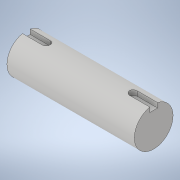
# Autodesk Inventor part: MotorShaft
Saved by Autodesk Inventor 2021 (Build 250183000, 183)
## iProperties
Created: 2020-09-20
Part Number: MotorShaft
Material: Generic
Document SubType Name: Modeling
Designer: PhotonUser
Density: 1 g/cm^3
Appearance: Default
Author: PhotonUser
Autodesk Inventor part; units mm, degrees
ref_plane "YZ Plane" through (0, 0, 0) normal (1, 0, 0) x (0, 1, 0)
ref_plane "XZ Plane" through (0, 0, 0) normal (0, 1, 0) x (-1, 0, 0)
ref_plane "XY Plane" through (0, 0, 0) normal (0, 0, 1) x (1, 0, 0)
sketch "Sketch1" plane through (0, 0, 0) normal (1, 0, 0) x (0, 1, 0)
  circle A0 centre (0, 0) radius 15.875
  dimension "d0" = 31.75
  constraints: 1 centre point, 1 coincident
  measures "d0" diameter of A0
extrude "Extrusion1" add sketch "Sketch1" along normal blind 104.3178
ref_plane "Work Plane1" through (52.1589, 0, 0) normal (1, 0, 0) x (0, 0, -1)
sketch "Sketch6" plane through (0, 0, 0) normal (-1, 0, 0) x (0, 0, 1)
  circle A0 centre (0, 0) radius 15.875 projected
  line L0 (-3.175, 15.5543) -> (-3.175, 11.7443)
  line L1 (-3.175, 11.7443) -> (3.175, 11.7443)
  line L2 (3.175, 11.7443) -> (3.175, 15.5543)
  arc A1 (3.175, 15.5543) -> (-3.175, 15.5543) centre (0, 0) ccw
  line L3 (0, 0) -> (0, 20.1314)
  point P0 (0, 11.7443)
  dimension "d16" = 3.81
  dimension "d17" = 6.35
  constraints: 8 end point, 4 point on circle, 2 vertical, 1 centre point, 1 coincident, 1 concentric, 1 horizontal, 1 midpoint, 1 perpendicular, 1 point on line
  measures "d16" distance of L0.start L0.end
  measures "d17" distance of L0.end L1.end
extrude "Extrusion6" cut sketch "Sketch6" against normal blind 16.51 contours L2 L1 L3 A0 | A0 L3 L1 L0
sketch "Sketch7" plane through (0, 11.7443, 3.175) normal (0, 1, 0) x (1, 0, 0)
  line L0 (0, 3.175) -> (25.5788, 3.175)
  line L1 (16.51, 0) -> (16.51, 6.35) projected
  line L2 (16.51, 7.6409) -> (16.51, 0)
  circle A0 centre (16.51, 3.175) radius 3.175
  constraints: 4 end point, 2 point on line, 1 collinear, 1 horizontal, 1 vertical alignment, 2 other
extrude "Extrusion7" cut sketch "Sketch7" along normal blind 19.05
mirror "Mirror2" about plane through (52.1589, 0, 0) normal (1, 0, 0) of "Extrusion6", "Extrusion7"
body "Solid1"
